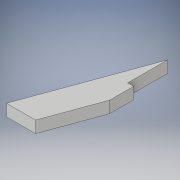
# Autodesk Inventor part: 2x4 leg stand
Saved by Autodesk Inventor 2019 (Build 230136000, 136)
## iProperties
Created: 2019-03-26
Part Number: 2x4 leg stand
Material: Generic
Document SubType Name: Modeling
Designer: torba
Density: 1 g/cm^3
Appearance: Default
Author: torba
Autodesk Inventor part; units mm, degrees
ref_plane "YZ Plane" through (0, 0, 0) normal (1, 0, 0) x (0, 1, 0)
ref_plane "XZ Plane" through (0, 0, 0) normal (0, 1, 0) x (-1, 0, 0)
ref_plane "XY Plane" through (0, 0, 0) normal (0, 0, 1) x (1, 0, 0)
sketch "Sketch1" plane through (0, 0, 0) normal (0, 1, 0) x (-1, 0, 0)
  line L0 (-11.0147, -115.5654) -> (128.7365, 268.3977)
  line L1 (-11.0147, -115.5654) -> (397.5903, -115.5654) construction
  line L2 (128.7365, 268.3977) -> (122.8702, 271.7846) construction
  line L3 (128.7365, 268.3977) -> (135.5103, 268.3977) construction
  line L4 (34.1311, 268.3977) -> (-30.0647, 92.0214)
  line L5 (122.8702, 271.7846) -> (685.799, 271.7846) construction
  line L6 (-30.0647, 14.3977) -> (-11.0147, 14.3977)
  line L7 (-30.0647, 14.3977) -> (-30.0647, 92.0214)
  line L8 (128.7365, 268.3977) -> (34.1311, 268.3977)
  line L9 (128.7365, 268.3977) -> (223.3419, 268.3977) construction
  line L10 (-11.0147, -115.5654) -> (-11.0147, 14.3977)
  dimension "d12" = 70
  dimension "d14" = 150
  dimension "d15" = 180
  dimension "d16" = 254
  dimension "d17" = 44.45
  dimension "d18" = 281.4644
  dimension "d19" = 387.35
  dimension "d20" = 19.05
  dimension "d22" = 88.9
  constraints: 22 end point, 4 horizontal, 3 equal length, 1 parallel, 1 perpendicular, 1 vertical
  measures "d12" angle of L1 L0
  measures "d14" angle of L3 L2
  measures "d15" angle of L8 L9
  measures "d16" distance between parallel lines of L6 L9
  measures "d17" distance from line of L6.end L4
  measures "d18" distance from line of L5.end L2
  measures "d19" distance between parallel lines of L5 L1
  measures "d20" distance between parallel lines of L7 L10
  measures "d22" distance between parallel lines of L4 L0
extrude "Extrusion1" add sketch "Sketch1" along normal blind 38.1
body "Solid1"
